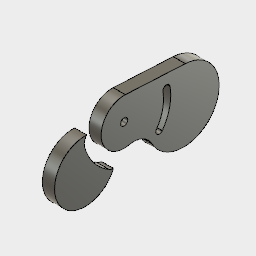
Chain Guide Nest (Autodesk Fusion 360 design; units mm, degrees)
Autodesk Fusion 360 part; units mm, degrees
sketch "Sketch1" plane through (0, 0, 0) normal (0, 0, 1) x (1, 0, 0) in component "Tensioner Mount Plate"
  line L0 (-29, 0) -> (29, 0)
  line L1 (-29, 0) -> (-29, -38.1)
  circle A0 centre (21, -30.1) radius 3.5
  line L2 (15.9481, -8.1745) -> (-41.2371, -21.3508)
  arc A1 (19.8875, -52.5725) -> (-0.1112, -66.3331) centre (18.8987, -72.548) ccw
  line L3 (29, -38.1) -> (29, 0)
  line L4 (-29, -38.1) -> (29, -38.1)
  line L5 (21, -30.1) -> (-21, -30.1) construction
  line L6 (21, -30.1) -> (-33.3785, -55.4571) construction
  line L7 (-21, -30.1) -> (-29, -30.1) construction
  line L8 (29, -30.1) -> (21, -30.1) construction
  arc A2 (-41.2371, -21.3508) -> (-0.1112, -66.3331) centre (-33.3785, -55.4571) ccw
  arc A3 (19.8875, -52.5725) -> (15.9481, -8.1745) centre (21, -30.1) ccw
  line L9 (21, -30.1) -> (-8.6985, -59.7985) construction
  arc A4 (-20.8635, -26.6027) -> (-6.129, -62.175) centre (21.248, -29.9973) ccw construction
  arc A5 (-17.5, -30.1) -> (-6.2236, -57.3236) centre (21, -30.1) ccw
  arc A6 (-24.5, -30.1) -> (-11.1734, -62.2734) centre (21, -30.1) ccw
  arc A7 (-11.1734, -62.2734) -> (-6.2236, -57.3236) centre (-8.6985, -59.7985) ccw
  arc A8 (-17.5, -30.1) -> (-24.5, -30.1) centre (-21, -30.1) ccw
  dimension "d56_1" = 8
  dimension "d57_1" = 8
  dimension "d58_1" = 7
  dimension "d59_1" = 45
  dimension "d60_1" = 35
  dimension "d61_1" = 20
  dimension "d63_1" = 60
  dimension "d64_1" = 25
  dimension "d65_1" = 45
  measures "d56_1" distance of A0.centre L3
  measures "d57_1" distance of A0.centre L4
  measures "d58_1" diameter of A0
  measures "d59_1" diameter of A3
  measures "d60_1" radius of A2
  measures "d61_1" radius of A1
  measures "d63_1" distance of A0.centre L6.end
  measures "d64_1" angle of L5 L6
  measures "d65_1" angle of L5 L9
extrude "Extrude1" add sketch "Sketch1" against normal blind 12 contours L1 L2 L3 L4 A3 A5 A6 A8 | L1 L2 A1 L3 L4 A2 A3 A5 A6 A7 makes body 1 in component "Tensioner Mount Plate"
sketch "Sketch2" plane through (0, 0, -12) normal (0, 0, -1) x (-1, 0, 0) in component "Tensioner"
  circle A0 centre (-21, -30.1) radius 3.5
  arc A1 (24.5, -30.1) -> (17.5, -30.1) centre (21, -30.1) ccw
  arc A2 (11.1734, -62.2734) -> (24.5, -30.1) centre (-21, -30.1) ccw
  arc A3 (6.2236, -57.3236) -> (11.1734, -62.2734) centre (8.6985, -59.7985) ccw
  arc A4 (6.2236, -57.3236) -> (17.5, -30.1) centre (-21, -30.1) ccw
  arc A5 (-15.9481, -8.1745) -> (-19.8875, -52.5725) centre (-21, -30.1) ccw
  arc A6 (0.1112, -66.3331) -> (-19.8875, -52.5725) centre (-18.8987, -72.548) ccw
  arc A7 (0.1112, -66.3331) -> (41.2371, -21.3508) centre (33.3785, -55.4571) ccw
  line L0 (41.2371, -21.3508) -> (-15.9481, -8.1745)
  arc A8 (11.1734, -62.2734) -> (24.5, -30.1) centre (-21, -30.1) ccw
  arc A9 (6.2236, -57.3236) -> (11.1734, -62.2734) centre (8.6985, -59.7985) ccw
  arc A10 (6.2236, -57.3236) -> (17.5, -30.1) centre (-21, -30.1) ccw
  arc A11 (24.5, -30.1) -> (17.5, -30.1) centre (21, -30.1) ccw
  arc A12 (0.1112, -66.3331) -> (41.2371, -21.3508) centre (33.3785, -55.4571) ccw
  line L1 (41.2371, -21.3508) -> (-15.9481, -8.1745)
  arc A13 (-15.9481, -8.1745) -> (-19.8875, -52.5725) centre (-21, -30.1) ccw
  arc A14 (0.1112, -66.3331) -> (-19.8875, -52.5725) centre (-18.8987, -72.548) ccw
  circle A15 centre (-21, -30.1) radius 3.5
  arc A16 (30.5, -30.1) -> (29.4291, -25.7182) centre (21, -30.1) ccw
  arc A17 (6.647, -69.0743) -> (15.416, -66.516) centre (8.6985, -59.7985) ccw
  arc A18 (15.416, -66.516) -> (30.5, -30.1) centre (-21, -30.1) ccw
  arc A19 (6.647, -69.0743) -> (29.4291, -25.7182) centre (33.3785, -55.4571) ccw
  dimension "d68_1" = 60
  measures "d68_1" diameter of A19
extrude "Extrude2" add sketch "Sketch2" along normal blind 12 separate body contours A16 A17 A18 A19 makes body 2 in component "Tensioner"
sketch "Sketch1 (2)" plane through (0, 0, 0) normal (1, 0, 0) x (0, 0, -1)
  line L0 (0, 0) -> (609, 0)
  line L1 (609, 0) -> (609, 609)
  line L2 (609, 609) -> (0, 609)
  line L3 (0, 609) -> (0, 0)
  dimension "d1" = 609
  dimension "d2" = 609
  measures "d1" distance of L0.start L0.end
  measures "d2" distance of L0.start L2.end
extrude "Extrude1'" add sketch "Sketch1 (2)" along normal blind 12 separate body makes body 3
component "Tensioner Mount Plate" placed x (0, -0.173648, 0.984808) y (0, 0.984808, 0.173648) z (-1, 0, 0) at (0, 98.8185, -97.4986)
component "Tensioner" placed x (0, 0.866025, -0.5) y (0, -0.5, -0.866025) z (-1, 0, 0) at (-12, 43.9643, -108.7618)
hidden bodies 3
